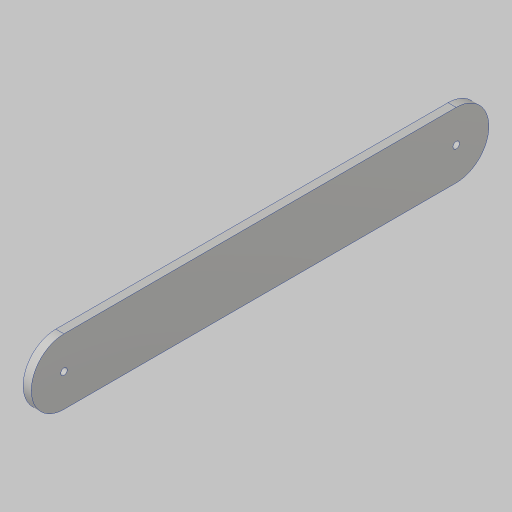
# Autodesk Inventor part: GI - 006
Saved by Autodesk Inventor 2023.5 (Build 275446000, 446)
## iProperties
Created: 2025-01-25
Part Number: GI - 006
Material: Aluminum 6061
Document SubType Name: Modeling
Designer: slick
Density: 2.7 g/cm^3
Appearance: Aluminum - Flat
Author: slick
Autodesk Inventor part; units mm, degrees
ref_plane "YZ Plane" through (0, 0, 0) normal (1, 0, 0) x (0, 1, 0)
ref_plane "XZ Plane" through (0, 0, 0) normal (0, 1, 0) x (-1, 0, 0)
ref_plane "XY Plane" through (0, 0, 0) normal (0, 0, 1) x (1, 0, 0)
sketch "Sketch1" plane through (0, 0, 0) normal (1, 0, 0) x (0, 1, 0)
  line L0 (0, -152.4) -> (0, 152.4) construction
  line L1 (25.4, -152.4) -> (25.4, 152.4)
  line L2 (-25.4, 152.4) -> (-25.4, -152.4)
  arc A0 (-25.4, -152.4) -> (25.4, -152.4) centre (0, -152.4) ccw
  arc A1 (25.4, 152.4) -> (-25.4, 152.4) centre (0, 152.4) ccw
  point P0 (0, 0)
  dimension "d0" = 50.8
  dimension "d1" = 304.8
  constraints: 8 end point, 4 point on circle, 4 tangent, 2 centre point, 2 coincident, 1 midpoint, 1 parallel, 1 vertical
  measures "d0" diameter of A1
  measures "d1" distance of L1.start L1.end
extrude "Extrusion1" add sketch "Sketch1" along normal blind 6.35
hole "Hole1" at (0, 0, 152.4) at (0, 0, -152.4) direction (1, 0, 0) diameter 5.1054 end through all clearance for "Flat Head Machine Screw (82)" size "#10" standard "Ansi Unified Screw Threads"
body "Solid1"
